Autodesk Inventor part; units mm, degrees
(part 3 of 6)
  line L1783 (-26.455, 14.4184) -> (-26.602, 14.5927)
  line L1784 (-26.602, 14.5927) -> (-26.7541, 14.7808)
  line L1785 (-26.7541, 14.7808) -> (-26.9091, 14.9811)
  line L1786 (-26.9091, 14.9811) -> (-27.041, 15.1586)
  arc A54 (-26.6482, 15.8389) -> (-27.041, 15.1586) centre (0, 0) ccw
  line L1787 (-26.6482, 15.8389) -> (-26.4285, 15.8134)
  line L1788 (-26.4285, 15.8134) -> (-26.1776, 15.7793)
  line L1789 (-26.1776, 15.7793) -> (-25.9387, 15.7417)
  line L1790 (-25.9387, 15.7417) -> (-25.7142, 15.7015)
  line L1791 (-25.7142, 15.7015) -> (-25.5018, 15.6589)
  line L1792 (-25.5018, 15.6589) -> (-25.3015, 15.6144)
  line L1793 (-25.3015, 15.6144) -> (-25.1161, 15.569)
  line L1794 (-25.1161, 15.569) -> (-24.9429, 15.5228)
  line L1795 (-24.9429, 15.5228) -> (-24.6058, 15.4237)
  line L1796 (-24.6058, 15.4237) -> (-24.5595, 15.4172)
  line L1797 (-24.5595, 15.4172) -> (-24.5238, 15.4191)
  line L1798 (-24.5238, 15.4191) -> (-24.4991, 15.4291)
  line L1799 (-24.4991, 15.4291) -> (-24.488, 15.4416)
  line L1800 (-24.488, 15.4416) -> (-24.2795, 15.7673)
  line L1801 (-24.2795, 15.7673) -> (-24.0668, 16.0903)
  line L1802 (-24.0668, 16.0903) -> (-24.0599, 16.1055)
  line L1803 (-24.0599, 16.1055) -> (-24.0608, 16.1321)
  line L1804 (-24.0608, 16.1321) -> (-24.0735, 16.1655)
  line L1805 (-24.0735, 16.1655) -> (-24.0984, 16.2052)
  line L1806 (-24.0984, 16.2052) -> (-24.326, 16.4728)
  line L1807 (-24.326, 16.4728) -> (-24.4386, 16.6122)
  line L1808 (-24.4386, 16.6122) -> (-24.5555, 16.7632)
  line L1809 (-24.5555, 16.7632) -> (-24.6777, 16.928)
  line L1810 (-24.6777, 16.928) -> (-24.8029, 17.1047)
  line L1811 (-24.8029, 17.1047) -> (-24.931, 17.2934)
  line L1812 (-24.931, 17.2934) -> (-25.0625, 17.4964)
  line L1813 (-25.0625, 17.4964) -> (-25.1957, 17.7118)
  line L1814 (-25.1957, 17.7118) -> (-25.3084, 17.9021)
  arc A55 (-24.8466, 18.5377) -> (-25.3084, 17.9021) centre (0, 0) ccw
  line L1815 (-24.8466, 18.5377) -> (-24.6308, 18.4893)
  line L1816 (-24.6308, 18.4893) -> (-24.3848, 18.4292)
  line L1817 (-24.3848, 18.4292) -> (-24.1511, 18.3668)
  line L1818 (-24.1511, 18.3668) -> (-23.932, 18.3034)
  line L1819 (-23.932, 18.3034) -> (-23.7253, 18.2388)
  line L1820 (-23.7253, 18.2388) -> (-23.5308, 18.1736)
  line L1821 (-23.5308, 18.1736) -> (-23.3511, 18.1091)
  line L1822 (-23.3511, 18.1091) -> (-23.1837, 18.045)
  line L1823 (-23.1837, 18.045) -> (-22.8588, 17.9112)
  line L1824 (-22.8588, 17.9112) -> (-22.8134, 17.8999)
  line L1825 (-22.8134, 17.8999) -> (-22.7777, 17.8981)
  line L1826 (-22.7777, 17.8981) -> (-22.7521, 17.9055)
  line L1827 (-22.7521, 17.9055) -> (-22.7398, 17.9167)
  line L1828 (-22.7398, 17.9167) -> (-22.4984, 18.2188)
  line L1829 (-22.4984, 18.2188) -> (-22.2531, 18.5178)
  line L1830 (-22.2531, 18.5178) -> (-22.2446, 18.5322)
  line L1831 (-22.2446, 18.5322) -> (-22.2427, 18.5587)
  line L1832 (-22.2427, 18.5587) -> (-22.2519, 18.5933)
  line L1833 (-22.2519, 18.5933) -> (-22.2724, 18.6353)
  line L1834 (-22.2724, 18.6353) -> (-22.4708, 18.9253)
  line L1835 (-22.4708, 18.9253) -> (-22.5683, 19.0757)
  line L1836 (-22.5683, 19.0757) -> (-22.6688, 19.2381)
  line L1837 (-22.6688, 19.2381) -> (-22.773, 19.4148)
  line L1838 (-22.773, 19.4148) -> (-22.8791, 19.6036)
  line L1839 (-22.8791, 19.6036) -> (-22.9867, 19.8047)
  line L1840 (-22.9867, 19.8047) -> (-23.0963, 20.0203)
  line L1841 (-23.0963, 20.0203) -> (-23.2063, 20.2484)
  line L1842 (-23.2063, 20.2484) -> (-23.2985, 20.4495)
  arc A56 (-22.7728, 21.0333) -> (-23.2985, 20.4495) centre (0, 0) ccw
  line L1843 (-22.7728, 21.0333) -> (-22.5632, 20.9626)
  line L1844 (-22.5632, 20.9626) -> (-22.3249, 20.8771)
  line L1845 (-22.3249, 20.8771) -> (-22.099, 20.7906)
  line L1846 (-22.099, 20.7906) -> (-21.8877, 20.7047)
  line L1847 (-21.8877, 20.7047) -> (-21.6889, 20.6189)
  line L1848 (-21.6889, 20.6189) -> (-21.5022, 20.5336)
  line L1849 (-21.5022, 20.5336) -> (-21.3302, 20.4507)
  line L1850 (-21.3302, 20.4507) -> (-21.1705, 20.3695)
  line L1851 (-21.1705, 20.3695) -> (-20.8614, 20.2025)
  line L1852 (-20.8614, 20.2025) -> (-20.8174, 20.1865)
  line L1853 (-20.8174, 20.1865) -> (-20.7821, 20.181)
  line L1854 (-20.7821, 20.181) -> (-20.7559, 20.1856)
  line L1855 (-20.7559, 20.1856) -> (-20.7424, 20.1955)
  line L1856 (-20.7424, 20.1955) -> (-20.4707, 20.4707)
  line L1857 (-20.4707, 20.4707) -> (-20.1955, 20.7424)
  line L1858 (-20.1955, 20.7424) -> (-20.1856, 20.7559)
  line L1859 (-20.1856, 20.7559) -> (-20.181, 20.7821)
  line L1860 (-20.181, 20.7821) -> (-20.1865, 20.8174)
  line L1861 (-20.1865, 20.8174) -> (-20.2025, 20.8614)
  line L1862 (-20.2025, 20.8614) -> (-20.3695, 21.1705)
  line L1863 (-20.3695, 21.1705) -> (-20.4507, 21.3302)
  line L1864 (-20.4507, 21.3302) -> (-20.5336, 21.5022)
  line L1865 (-20.5336, 21.5022) -> (-20.6189, 21.6889)
  line L1866 (-20.6189, 21.6889) -> (-20.7047, 21.8877)
  line L1867 (-20.7047, 21.8877) -> (-20.7906, 22.099)
  line L1868 (-20.7906, 22.099) -> (-20.8771, 22.3249)
  line L1869 (-20.8771, 22.3249) -> (-20.9626, 22.5632)
  line L1870 (-20.9626, 22.5632) -> (-21.0333, 22.7728)
  arc A57 (-20.4495, 23.2985) -> (-21.0333, 22.7728) centre (0, 0) ccw
  line L1871 (-20.4495, 23.2985) -> (-20.2484, 23.2063)
  line L1872 (-20.2484, 23.2063) -> (-20.0203, 23.0963)
  line L1873 (-20.0203, 23.0963) -> (-19.8047, 22.9867)
  line L1874 (-19.8047, 22.9867) -> (-19.6036, 22.8791)
  line L1875 (-19.6036, 22.8791) -> (-19.4148, 22.773)
  line L1876 (-19.4148, 22.773) -> (-19.2381, 22.6688)
  line L1877 (-19.2381, 22.6688) -> (-19.0757, 22.5683)
  line L1878 (-19.0757, 22.5683) -> (-18.9253, 22.4708)
  line L1879 (-18.9253, 22.4708) -> (-18.6353, 22.2724)
  line L1880 (-18.6353, 22.2724) -> (-18.5933, 22.2519)
  line L1881 (-18.5933, 22.2519) -> (-18.5587, 22.2427)
  line L1882 (-18.5587, 22.2427) -> (-18.5322, 22.2446)
  line L1883 (-18.5322, 22.2446) -> (-18.5178, 22.2531)
  line L1884 (-18.5178, 22.2531) -> (-18.2188, 22.4984)
  line L1885 (-18.2188, 22.4984) -> (-17.9167, 22.7398)
  line L1886 (-17.9167, 22.7398) -> (-17.9055, 22.7521)
  line L1887 (-17.9055, 22.7521) -> (-17.8981, 22.7777)
  line L1888 (-17.8981, 22.7777) -> (-17.8999, 22.8134)
  line L1889 (-17.8999, 22.8134) -> (-17.9112, 22.8588)
  line L1890 (-17.9112, 22.8588) -> (-18.045, 23.1837)
  line L1891 (-18.045, 23.1837) -> (-18.1091, 23.3511)
  line L1892 (-18.1091, 23.3511) -> (-18.1736, 23.5308)
  line L1893 (-18.1736, 23.5308) -> (-18.2388, 23.7253)
  line L1894 (-18.2388, 23.7253) -> (-18.3034, 23.932)
  line L1895 (-18.3034, 23.932) -> (-18.3668, 24.1511)
  line L1896 (-18.3668, 24.1511) -> (-18.4292, 24.3848)
  line L1897 (-18.4292, 24.3848) -> (-18.4893, 24.6308)
  line L1898 (-18.4893, 24.6308) -> (-18.5377, 24.8466)
  arc A58 (-17.9021, 25.3084) -> (-18.5377, 24.8466) centre (0, 0) ccw
  line L1899 (-17.9021, 25.3084) -> (-17.7118, 25.1957)
  line L1900 (-17.7118, 25.1957) -> (-17.4964, 25.0625)
  line L1901 (-17.4964, 25.0625) -> (-17.2934, 24.931)
  line L1902 (-17.2934, 24.931) -> (-17.1047, 24.8029)
  line L1903 (-17.1047, 24.8029) -> (-16.928, 24.6777)
  line L1904 (-16.928, 24.6777) -> (-16.7632, 24.5555)
  line L1905 (-16.7632, 24.5555) -> (-16.6122, 24.4386)
  line L1906 (-16.6122, 24.4386) -> (-16.4728, 24.326)
  line L1907 (-16.4728, 24.326) -> (-16.2052, 24.0984)
  line L1908 (-16.2052, 24.0984) -> (-16.1655, 24.0735)
  line L1909 (-16.1655, 24.0735) -> (-16.1321, 24.0608)
  line L1910 (-16.1321, 24.0608) -> (-16.1055, 24.0599)
  line L1911 (-16.1055, 24.0599) -> (-16.0903, 24.0668)
  line L1912 (-16.0903, 24.0668) -> (-15.7673, 24.2795)
  line L1913 (-15.7673, 24.2795) -> (-15.4416, 24.488)
  line L1914 (-15.4416, 24.488) -> (-15.4291, 24.4991)
  line L1915 (-15.4291, 24.4991) -> (-15.4191, 24.5238)
  line L1916 (-15.4191, 24.5238) -> (-15.4172, 24.5595)
  line L1917 (-15.4172, 24.5595) -> (-15.4237, 24.6058)
  line L1918 (-15.4237, 24.6058) -> (-15.5228, 24.9429)
  line L1919 (-15.5228, 24.9429) -> (-15.569, 25.1161)
  line L1920 (-15.569, 25.1161) -> (-15.6144, 25.3015)
  line L1921 (-15.6144, 25.3015) -> (-15.6589, 25.5018)
  line L1922 (-15.6589, 25.5018) -> (-15.7015, 25.7142)
  line L1923 (-15.7015, 25.7142) -> (-15.7417, 25.9387)
  line L1924 (-15.7417, 25.9387) -> (-15.7793, 26.1776)
  line L1925 (-15.7793, 26.1776) -> (-15.8134, 26.4285)
  line L1926 (-15.8134, 26.4285) -> (-15.8389, 26.6482)
  arc A59 (-15.1586, 27.041) -> (-15.8389, 26.6482) centre (0, 0) ccw
  line L1927 (-15.1586, 27.041) -> (-14.9811, 26.9091)
  line L1928 (-14.9811, 26.9091) -> (-14.7808, 26.7541)
  line L1929 (-14.7808, 26.7541) -> (-14.5927, 26.602)
  line L1930 (-14.5927, 26.602) -> (-14.4184, 26.455)
  line L1931 (-14.4184, 26.455) -> (-14.2558, 26.312)
  line L1932 (-14.2558, 26.312) -> (-14.1046, 26.1732)
  line L1933 (-14.1046, 26.1732) -> (-13.9666, 26.0412)
  line L1934 (-13.9666, 26.0412) -> (-13.8398, 25.9146)
  line L1935 (-13.8398, 25.9146) -> (-13.5974, 25.6603)
  line L1936 (-13.5974, 25.6603) -> (-13.5605, 25.6314)
  line L1937 (-13.5605, 25.6314) -> (-13.5287, 25.6153)
  line L1938 (-13.5287, 25.6153) -> (-13.5023, 25.6116)
  line L1939 (-13.5023, 25.6116) -> (-13.4865, 25.6168)
  line L1940 (-13.4865, 25.6168) -> (-13.143, 25.7946)
  line L1941 (-13.143, 25.7946) -> (-12.7973, 25.968)
  line L1942 (-12.7973, 25.968) -> (-12.7837, 25.9777)
  line L1943 (-12.7837, 25.9777) -> (-12.7712, 26.0012)
  line L1944 (-12.7712, 26.0012) -> (-12.7656, 26.0365)
  line L1945 (-12.7656, 26.0365) -> (-12.7672, 26.0833)
  line L1946 (-12.7672, 26.0833) -> (-12.8305, 26.4288)
  line L1947 (-12.8305, 26.4288) -> (-12.8584, 26.6059)
  line L1948 (-12.8584, 26.6059) -> (-12.8841, 26.7951)
  line L1949 (-12.8841, 26.7951) -> (-12.9075, 26.9989)
  line L1950 (-12.9075, 26.9989) -> (-12.9276, 27.2145)
  line L1951 (-12.9276, 27.2145) -> (-12.9441, 27.442)
  line L1952 (-12.9441, 27.442) -> (-12.9565, 27.6836)
  line L1953 (-12.9565, 27.6836) -> (-12.9642, 27.9367)
  line L1954 (-12.9642, 27.9367) -> (-12.9667, 28.1579)
  arc A60 (-12.249, 28.4774) -> (-12.9667, 28.1579) centre (0, 0) ccw
  line L1955 (-12.249, 28.4774) -> (-12.0862, 28.3276)
  line L1956 (-12.0862, 28.3276) -> (-11.9033, 28.1525)
  line L1957 (-11.9033, 28.1525) -> (-11.7321, 27.9817)
  line L1958 (-11.7321, 27.9817) -> (-11.5741, 27.8172)
  line L1959 (-11.5741, 27.8172) -> (-11.4273, 27.6579)
  line L1960 (-11.4273, 27.6579) -> (-11.2915, 27.5042)
  line L1961 (-11.2915, 27.5042) -> (-11.1681, 27.3584)
  line L1962 (-11.1681, 27.3584) -> (-11.0551, 27.2193)
  line L1963 (-11.0551, 27.2193) -> (-10.8407, 26.941)
  line L1964 (-10.8407, 26.941) -> (-10.807, 26.9085)
  line L1965 (-10.807, 26.9085) -> (-10.777, 26.8891)
  line L1966 (-10.777, 26.8891) -> (-10.7512, 26.8826)
  line L1967 (-10.7512, 26.8826) -> (-10.7349, 26.8862)
  line L1968 (-10.7349, 26.8862) -> (-10.3748, 27.0272)
  line L1969 (-10.3748, 27.0272) -> (-10.0128, 27.1634)
  line L1970 (-10.0128, 27.1634) -> (-9.9983, 27.1717)
  line L1971 (-9.9983, 27.1717) -> (-9.9834, 27.1937)
  line L1972 (-9.9834, 27.1937) -> (-9.9741, 27.2282)
  line L1973 (-9.9741, 27.2282) -> (-9.9708, 27.2749)
  line L1974 (-9.9708, 27.2749) -> (-9.9977, 27.6252)
  line L1975 (-9.9977, 27.6252) -> (-10.0069, 27.8042)
  line L1976 (-10.0069, 27.8042) -> (-10.0127, 27.995)
  line L1977 (-10.0127, 27.995) -> (-10.0146, 28.2002)
  line L1978 (-10.0146, 28.2002) -> (-10.0121, 28.4168)
  line L1979 (-10.0121, 28.4168) -> (-10.0047, 28.6447)
  line L1980 (-10.0047, 28.6447) -> (-9.9918, 28.8863)
  line L1981 (-9.9918, 28.8863) -> (-9.973, 29.1388)
  line L1982 (-9.973, 29.1388) -> (-9.9523, 29.359)
  arc A61 (-9.2052, 29.6018) -> (-9.9523, 29.359) centre (0, 0) ccw
  line L1983 (-9.2052, 29.6018) -> (-9.059, 29.4358)
  line L1984 (-9.059, 29.4358) -> (-8.8954, 29.2425)
  line L1985 (-8.8954, 29.2425) -> (-8.7429, 29.0547)
  line L1986 (-8.7429, 29.0547) -> (-8.603, 28.8746)
  line L1987 (-8.603, 28.8746) -> (-8.4737, 28.7009)
  line L1988 (-8.4737, 28.7009) -> (-8.3547, 28.5338)
  line L1989 (-8.3547, 28.5338) -> (-8.2472, 28.3759)
  line L1990 (-8.2472, 28.3759) -> (-8.1494, 28.2257)
  line L1991 (-8.1494, 28.2257) -> (-7.9652, 27.9266)
  line L1992 (-7.9652, 27.9266) -> (-7.9351, 27.8907)
  line L1993 (-7.9351, 27.8907) -> (-7.9073, 27.8683)
  line L1994 (-7.9073, 27.8683) -> (-7.8823, 27.8592)
  line L1995 (-7.8823, 27.8592) -> (-7.8657, 27.861)
  line L1996 (-7.8657, 27.861) -> (-7.4928, 27.9636)
  line L1997 (-7.4928, 27.9636) -> (-7.1186, 28.0612)
  line L1998 (-7.1186, 28.0612) -> (-7.1033, 28.0679)
  line L1999 (-7.1033, 28.0679) -> (-7.0862, 28.0883)
  line L2000 (-7.0862, 28.0883) -> (-7.0733, 28.1216)
  line L2001 (-7.0733, 28.1216) -> (-7.0652, 28.1677)
  line L2002 (-7.0652, 28.1677) -> (-7.0553, 28.5189)
  line L2003 (-7.0553, 28.5189) -> (-7.0457, 28.6979)
  line L2004 (-7.0457, 28.6979) -> (-7.0315, 28.8883)
  line L2005 (-7.0315, 28.8883) -> (-7.012, 29.0926)
  line L2006 (-7.012, 29.0926) -> (-6.9869, 29.3077)
  line L2007 (-6.9869, 29.3077) -> (-6.9557, 29.5336)
  line L2008 (-6.9557, 29.5336) -> (-6.9177, 29.7725)
  line L2009 (-6.9177, 29.7725) -> (-6.8726, 30.0216)
  line L2010 (-6.8726, 30.0216) -> (-6.829, 30.2385)
  arc A62 (-6.0605, 30.4018) -> (-6.829, 30.2385) centre (0, 0) ccw
  line L2011 (-6.0605, 30.4018) -> (-5.9325, 30.2214)
  line L2012 (-5.9325, 30.2214) -> (-5.79, 30.0122)
  line L2013 (-5.79, 30.0122) -> (-5.658, 29.8094)
  line L2014 (-5.658, 29.8094) -> (-5.5376, 29.6157)
  line L2015 (-5.5376, 29.6157) -> (-5.4272, 29.4294)
  line L2016 (-5.4272, 29.4294) -> (-5.3263, 29.2508)
  line L2017 (-5.3263, 29.2508) -> (-5.2359, 29.0826)
  line L2018 (-5.2359, 29.0826) -> (-5.1544, 28.9229)
  line L2019 (-5.1544, 28.9229) -> (-5.0025, 28.6062)
  line L2020 (-5.0025, 28.6062) -> (-4.9763, 28.5674)
  line L2021 (-4.9763, 28.5674) -> (-4.951, 28.5421)
  line L2022 (-4.951, 28.5421) -> (-4.927, 28.5305)
  line L2023 (-4.927, 28.5305) -> (-4.9104, 28.5306)
  line L2024 (-4.9104, 28.5306) -> (-4.5288, 28.5936)
  line L2025 (-4.5288, 28.5936) -> (-4.1464, 28.6516)
  line L2026 (-4.1464, 28.6516) -> (-4.1305, 28.6567)
  line L2027 (-4.1305, 28.6567) -> (-4.1114, 28.6751)
  line L2028 (-4.1114, 28.6751) -> (-4.0951, 28.7069)
  line L2029 (-4.0951, 28.7069) -> (-4.0822, 28.7519)
  line L2030 (-4.0822, 28.7519) -> (-4.0356, 29.1001)
  line L2031 (-4.0356, 29.1001) -> (-4.0074, 29.2771)
  line L2032 (-4.0074, 29.2771) -> (-3.9734, 29.465)
  line L2033 (-3.9734, 29.465) -> (-3.9326, 29.6661)
  line L2034 (-3.9326, 29.6661) -> (-3.8852, 29.8774)
  line L2035 (-3.8852, 29.8774) -> (-3.8305, 30.0989)
  line L2036 (-3.8305, 30.0989) -> (-3.7677, 30.3325)
  line L2037 (-3.7677, 30.3325) -> (-3.6968, 30.5755)
  line L2038 (-3.6968, 30.5755) -> (-3.6308, 30.7866)
  arc A63 (-2.8495, 30.8688) -> (-3.6308, 30.7866) centre (0, 0) ccw
  line L2039 (-2.8495, 30.8688) -> (-2.741, 30.676)
  line L2040 (-2.741, 30.676) -> (-2.6211, 30.453)
  line L2041 (-2.6211, 30.453) -> (-2.5111, 30.2376)
  line L2042 (-2.5111, 30.2376) -> (-2.4116, 30.0323)
  line L2043 (-2.4116, 30.0323) -> (-2.3213, 29.8355)
  line L2044 (-2.3213, 29.8355) -> (-2.2396, 29.6473)
  line L2045 (-2.2396, 29.6473) -> (-2.1673, 29.4705)
  line L2046 (-2.1673, 29.4705) -> (-2.1029, 29.3033)
  line L2047 (-2.1029, 29.3033) -> (-1.9849, 28.9724)
  line L2048 (-1.9849, 28.9724) -> (-1.9629, 28.931)
  line L2049 (-1.9629, 28.931) -> (-1.9404, 28.9033)
  line L2050 (-1.9404, 28.9033) -> (-1.9178, 28.8892)
  line L2051 (-1.9178, 28.8892) -> (-1.9012, 28.8876)
  line L2052 (-1.9012, 28.8876) -> (-1.5151, 28.9103)
  line L2053 (-1.5151, 28.9103) -> (-1.1288, 28.9281)
  line L2054 (-1.1288, 28.9281) -> (-1.1124, 28.9314)
  line L2055 (-1.1124, 28.9314) -> (-1.0915, 28.9478)
  line L2056 (-1.0915, 28.9478) -> (-1.0719, 28.9777)
  line L2057 (-1.0719, 28.9777) -> (-1.0544, 29.0211)
  line L2058 (-1.0544, 29.0211) -> (-0.9717, 29.3626)
  line L2059 (-0.9717, 29.3626) -> (-0.9251, 29.5356)
  line L2060 (-0.9251, 29.5356) -> (-0.8717, 29.719)
  line L2061 (-0.8717, 29.719) -> (-0.8101, 29.9147)
  line L2062 (-0.8101, 29.9147) -> (-0.7408, 30.1199)
  line L2063 (-0.7408, 30.1199) -> (-0.6634, 30.3344)
  line L2064 (-0.6634, 30.3344) -> (-0.5765, 30.5601)
  line L2065 (-0.5765, 30.5601) -> (-0.4805, 30.7945)
  line L2066 (-0.4805, 30.7945) -> (-0.3928, 30.9975)
  arc A64 (0.3928, 30.9975) -> (-0.3928, 30.9975) centre (0, 0) ccw
  line L2067 (0.3928, 30.9975) -> (0.4805, 30.7945)
  line L2068 (0.4805, 30.7945) -> (0.5765, 30.5601)
  line L2069 (0.5765, 30.5601) -> (0.6634, 30.3344)
  line L2070 (0.6634, 30.3344) -> (0.7408, 30.1199)
  line L2071 (0.7408, 30.1199) -> (0.8101, 29.9147)
  line L2072 (0.8101, 29.9147) -> (0.8717, 29.719)
  line L2073 (0.8717, 29.719) -> (0.9251, 29.5356)
  line L2074 (0.9251, 29.5356) -> (0.9717, 29.3626)
  line L2075 (0.9717, 29.3626) -> (1.0544, 29.0211)
  line L2076 (1.0544, 29.0211) -> (1.0719, 28.9777)
  line L2077 (1.0719, 28.9777) -> (1.0915, 28.9478)
  line L2078 (1.0915, 28.9478) -> (1.1124, 28.9314)
  line L2079 (1.1124, 28.9314) -> (1.1288, 28.9281)
  line L2080 (1.1288, 28.9281) -> (1.5151, 28.9103)
  line L2081 (1.5151, 28.9103) -> (1.9012, 28.8876)
  line L2082 (1.9012, 28.8876) -> (1.9178, 28.8892)
  line L2083 (1.9178, 28.8892) -> (1.9404, 28.9033)
  line L2084 (1.9404, 28.9033) -> (1.9629, 28.931)
  line L2085 (1.9629, 28.931) -> (1.9849, 28.9724)
  line L2086 (1.9849, 28.9724) -> (2.1029, 29.3033)
  line L2087 (2.1029, 29.3033) -> (2.1673, 29.4705)
  line L2088 (2.1673, 29.4705) -> (2.2396, 29.6473)
  line L2089 (2.2396, 29.6473) -> (2.3213, 29.8355)
  line L2090 (2.3213, 29.8355) -> (2.4116, 30.0323)
  line L2091 (2.4116, 30.0323) -> (2.5111, 30.2376)
  line L2092 (2.5111, 30.2376) -> (2.6211, 30.453)
  line L2093 (2.6211, 30.453) -> (2.741, 30.676)
  line L2094 (2.741, 30.676) -> (2.8495, 30.8688)
  arc A65 (3.6308, 30.7866) -> (2.8495, 30.8688) centre (0, 0) ccw
  line L2095 (3.6308, 30.7866) -> (3.6968, 30.5755)
  line L2096 (3.6968, 30.5755) -> (3.7677, 30.3325)
  line L2097 (3.7677, 30.3325) -> (3.8305, 30.0989)
  line L2098 (3.8305, 30.0989) -> (3.8852, 29.8774)
  line L2099 (3.8852, 29.8774) -> (3.9326, 29.6661)
  line L2100 (3.9326, 29.6661) -> (3.9734, 29.465)
  line L2101 (3.9734, 29.465) -> (4.0074, 29.2771)
  line L2102 (4.0074, 29.2771) -> (4.0356, 29.1001)
  line L2103 (4.0356, 29.1001) -> (4.0822, 28.7519)
  line L2104 (4.0822, 28.7519) -> (4.0951, 28.7069)
  line L2105 (4.0951, 28.7069) -> (4.1114, 28.6751)
  line L2106 (4.1114, 28.6751) -> (4.1305, 28.6567)
  line L2107 (4.1305, 28.6567) -> (4.1464, 28.6516)
  line L2108 (4.1464, 28.6516) -> (4.5288, 28.5936)
  line L2109 (4.5288, 28.5936) -> (4.9104, 28.5306)
  line L2110 (4.9104, 28.5306) -> (4.927, 28.5305)
  line L2111 (4.927, 28.5305) -> (4.951, 28.5421)
  line L2112 (4.951, 28.5421) -> (4.9763, 28.5674)
  line L2113 (4.9763, 28.5674) -> (5.0025, 28.6062)
  line L2114 (5.0025, 28.6062) -> (5.1544, 28.9229)
  line L2115 (5.1544, 28.9229) -> (5.2359, 29.0826)
  line L2116 (5.2359, 29.0826) -> (5.3263, 29.2508)
  line L2117 (5.3263, 29.2508) -> (5.4272, 29.4294)
  line L2118 (5.4272, 29.4294) -> (5.5376, 29.6157)
  line L2119 (5.5376, 29.6157) -> (5.658, 29.8094)
  line L2120 (5.658, 29.8094) -> (5.79, 30.0122)
  line L2121 (5.79, 30.0122) -> (5.9325, 30.2214)
  line L2122 (5.9325, 30.2214) -> (6.0605, 30.4018)
  arc A66 (6.829, 30.2385) -> (6.0605, 30.4018) centre (0, 0) ccw
  line L2123 (6.829, 30.2385) -> (6.8726, 30.0216)
  line L2124 (6.8726, 30.0216) -> (6.9177, 29.7725)
  line L2125 (6.9177, 29.7725) -> (6.9557, 29.5336)
  line L2126 (6.9557, 29.5336) -> (6.9869, 29.3077)
  line L2127 (6.9869, 29.3077) -> (7.012, 29.0926)
  line L2128 (7.012, 29.0926) -> (7.0315, 28.8883)
  line L2129 (7.0315, 28.8883) -> (7.0457, 28.6979)
  line L2130 (7.0457, 28.6979) -> (7.0553, 28.5189)
  line L2131 (7.0553, 28.5189) -> (7.0652, 28.1677)
  line L2132 (7.0652, 28.1677) -> (7.0733, 28.1216)
  line L2133 (7.0733, 28.1216) -> (7.0862, 28.0883)
  line L2134 (7.0862, 28.0883) -> (7.1033, 28.0679)
  line L2135 (7.1033, 28.0679) -> (7.1186, 28.0612)
  line L2136 (7.1186, 28.0612) -> (7.4928, 27.9636)
  line L2137 (7.4928, 27.9636) -> (7.8657, 27.861)
  line L2138 (7.8657, 27.861) -> (7.8823, 27.8592)
  line L2139 (7.8823, 27.8592) -> (7.9073, 27.8683)
  line L2140 (7.9073, 27.8683) -> (7.9351, 27.8907)
  line L2141 (7.9351, 27.8907) -> (7.9652, 27.9266)
  line L2142 (7.9652, 27.9266) -> (8.1494, 28.2257)
  line L2143 (8.1494, 28.2257) -> (8.2472, 28.3759)
  line L2144 (8.2472, 28.3759) -> (8.3547, 28.5338)
  line L2145 (8.3547, 28.5338) -> (8.4737, 28.7009)
  line L2146 (8.4737, 28.7009) -> (8.603, 28.8746)
  line L2147 (8.603, 28.8746) -> (8.7429, 29.0547)
  line L2148 (8.7429, 29.0547) -> (8.8954, 29.2425)
  line L2149 (8.8954, 29.2425) -> (9.059, 29.4358)
  line L2150 (9.059, 29.4358) -> (9.2052, 29.6018)
  arc A67 (9.9523, 29.359) -> (9.2052, 29.6018) centre (0, 0) ccw
  line L2151 (9.9523, 29.359) -> (9.973, 29.1388)
  line L2152 (9.973, 29.1388) -> (9.9918, 28.8863)
  line L2153 (9.9918, 28.8863) -> (10.0047, 28.6447)
  line L2154 (10.0047, 28.6447) -> (10.0121, 28.4168)
  line L2155 (10.0121, 28.4168) -> (10.0146, 28.2002)
  line L2156 (10.0146, 28.2002) -> (10.0127, 27.995)
  line L2157 (10.0127, 27.995) -> (10.0069, 27.8042)
  line L2158 (10.0069, 27.8042) -> (9.9977, 27.6252)
  line L2159 (9.9977, 27.6252) -> (9.9708, 27.2749)
  line L2160 (9.9708, 27.2749) -> (9.9741, 27.2282)
  line L2161 (9.9741, 27.2282) -> (9.9834, 27.1937)
  line L2162 (9.9834, 27.1937) -> (9.9983, 27.1717)
  line L2163 (9.9983, 27.1717) -> (10.0128, 27.1634)
  line L2164 (10.0128, 27.1634) -> (10.3748, 27.0272)
  line L2165 (10.3748, 27.0272) -> (10.7349, 26.8862)
  line L2166 (10.7349, 26.8862) -> (10.7512, 26.8826)
  line L2167 (10.7512, 26.8826) -> (10.777, 26.8891)
  line L2168 (10.777, 26.8891) -> (10.807, 26.9085)
  line L2169 (10.807, 26.9085) -> (10.8407, 26.941)
  line L2170 (10.8407, 26.941) -> (11.0551, 27.2193)
  line L2171 (11.0551, 27.2193) -> (11.1681, 27.3584)
  line L2172 (11.1681, 27.3584) -> (11.2915, 27.5042)
  line L2173 (11.2915, 27.5042) -> (11.4273, 27.6579)
  line L2174 (11.4273, 27.6579) -> (11.5741, 27.8172)
  line L2175 (11.5741, 27.8172) -> (11.7321, 27.9817)
  line L2176 (11.7321, 27.9817) -> (11.9033, 28.1525)
  line L2177 (11.9033, 28.1525) -> (12.0862, 28.3276)
  line L2178 (12.0862, 28.3276) -> (12.249, 28.4774)
  arc A68 (12.9667, 28.1579) -> (12.249, 28.4774) centre (0, 0) ccw
  line L2179 (12.9667, 28.1579) -> (12.9642, 27.9367)
  line L2180 (12.9642, 27.9367) -> (12.9565, 27.6836)
  line L2181 (12.9565, 27.6836) -> (12.9441, 27.442)
  line L2182 (12.9441, 27.442) -> (12.9276, 27.2145)
  line L2183 (12.9276, 27.2145) -> (12.9075, 26.9989)
  line L2184 (12.9075, 26.9989) -> (12.8841, 26.7951)
  line L2185 (12.8841, 26.7951) -> (12.8584, 26.6059)
  line L2186 (12.8584, 26.6059) -> (12.8305, 26.4288)
  line L2187 (12.8305, 26.4288) -> (12.7672, 26.0833)
  line L2188 (12.7672, 26.0833) -> (12.7656, 26.0365)
  line L2189 (12.7656, 26.0365) -> (12.7712, 26.0012)
  line L2190 (12.7712, 26.0012) -> (12.7837, 25.9777)
  line L2191 (12.7837, 25.9777) -> (12.7973, 25.968)
  line L2192 (12.7973, 25.968) -> (13.143, 25.7946)
  line L2193 (13.143, 25.7946) -> (13.4865, 25.6168)
  line L2194 (13.4865, 25.6168) -> (13.5023, 25.6116)
  line L2195 (13.5023, 25.6116) -> (13.5287, 25.6153)
  line L2196 (13.5287, 25.6153) -> (13.5605, 25.6314)
  line L2197 (13.5605, 25.6314) -> (13.5974, 25.6603)
  line L2198 (13.5974, 25.6603) -> (13.8398, 25.9146)
  line L2199 (13.8398, 25.9146) -> (13.9666, 26.0412)
  line L2200 (13.9666, 26.0412) -> (14.1046, 26.1732)
  line L2201 (14.1046, 26.1732) -> (14.2558, 26.312)
  line L2202 (14.2558, 26.312) -> (14.4184, 26.455)
  line L2203 (14.4184, 26.455) -> (14.5927, 26.602)
  line L2204 (14.5927, 26.602) -> (14.7808, 26.7541)
  line L2205 (14.7808, 26.7541) -> (14.9811, 26.9091)
  line L2206 (14.9811, 26.9091) -> (15.1586, 27.041)
  arc A69 (15.8389, 26.6482) -> (15.1586, 27.041) centre (0, 0) ccw
  line L2207 (15.8389, 26.6482) -> (15.8134, 26.4285)
  line L2208 (15.8134, 26.4285) -> (15.7793, 26.1776)
  line L2209 (15.7793, 26.1776) -> (15.7417, 25.9387)
  line L2210 (15.7417, 25.9387) -> (15.7015, 25.7142)
  line L2211 (15.7015, 25.7142) -> (15.6589, 25.5018)
  line L2212 (15.6589, 25.5018) -> (15.6144, 25.3015)
  line L2213 (15.6144, 25.3015) -> (15.569, 25.1161)
  line L2214 (15.569, 25.1161) -> (15.5228, 24.9429)
  line L2215 (15.5228, 24.9429) -> (15.4237, 24.6058)
  line L2216 (15.4237, 24.6058) -> (15.4172, 24.5595)
  line L2217 (15.4172, 24.5595) -> (15.4191, 24.5238)
  line L2218 (15.4191, 24.5238) -> (15.4291, 24.4991)
  line L2219 (15.4291, 24.4991) -> (15.4416, 24.488)
  line L2220 (15.4416, 24.488) -> (15.7673, 24.2795)
  line L2221 (15.7673, 24.2795) -> (16.0903, 24.0668)
  line L2222 (16.0903, 24.0668) -> (16.1055, 24.0599)
  line L2223 (16.1055, 24.0599) -> (16.1321, 24.0608)
  line L2224 (16.1321, 24.0608) -> (16.1655, 24.0735)
  line L2225 (16.1655, 24.0735) -> (16.2052, 24.0984)
  line L2226 (16.2052, 24.0984) -> (16.4728, 24.326)
  line L2227 (16.4728, 24.326) -> (16.6122, 24.4386)
  line L2228 (16.6122, 24.4386) -> (16.7632, 24.5555)
  line L2229 (16.7632, 24.5555) -> (16.928, 24.6777)
  line L2230 (16.928, 24.6777) -> (17.1047, 24.8029)
  line L2231 (17.1047, 24.8029) -> (17.2934, 24.931)
  line L2232 (17.2934, 24.931) -> (17.4964, 25.0625)
  line L2233 (17.4964, 25.0625) -> (17.7118, 25.1957)
  line L2234 (17.7118, 25.1957) -> (17.9021, 25.3084)
  arc A70 (18.5377, 24.8466) -> (17.9021, 25.3084) centre (0, 0) ccw
  line L2235 (18.5377, 24.8466) -> (18.4893, 24.6308)
  line L2236 (18.4893, 24.6308) -> (18.4292, 24.3848)
  line L2237 (18.4292, 24.3848) -> (18.3668, 24.1511)
  line L2238 (18.3668, 24.1511) -> (18.3034, 23.932)
  line L2239 (18.3034, 23.932) -> (18.2388, 23.7253)
  line L2240 (18.2388, 23.7253) -> (18.1736, 23.5308)
  line L2241 (18.1736, 23.5308) -> (18.1091, 23.3511)
  line L2242 (18.1091, 23.3511) -> (18.045, 23.1837)
  line L2243 (18.045, 23.1837) -> (17.9112, 22.8588)
  line L2244 (17.9112, 22.8588) -> (17.8999, 22.8134)
  line L2245 (17.8999, 22.8134) -> (17.8981, 22.7777)
  line L2246 (17.8981, 22.7777) -> (17.9055, 22.7521)
  line L2247 (17.9055, 22.7521) -> (17.9167, 22.7398)
  line L2248 (17.9167, 22.7398) -> (18.2188, 22.4984)
  line L2249 (18.2188, 22.4984) -> (18.5178, 22.2531)
  line L2250 (18.5178, 22.2531) -> (18.5322, 22.2446)
  line L2251 (18.5322, 22.2446) -> (18.5587, 22.2427)
  line L2252 (18.5587, 22.2427) -> (18.5933, 22.2519)
  line L2253 (18.5933, 22.2519) -> (18.6353, 22.2724)
  line L2254 (18.6353, 22.2724) -> (18.9253, 22.4708)
  line L2255 (18.9253, 22.4708) -> (19.0757, 22.5683)
  line L2256 (19.0757, 22.5683) -> (19.2381, 22.6688)
  line L2257 (19.2381, 22.6688) -> (19.4148, 22.773)
  line L2258 (19.4148, 22.773) -> (19.6036, 22.8791)
  line L2259 (19.6036, 22.8791) -> (19.8047, 22.9867)
  line L2260 (19.8047, 22.9867) -> (20.0203, 23.0963)
  line L2261 (20.0203, 23.0963) -> (20.2484, 23.2063)
  line L2262 (20.2484, 23.2063) -> (20.4495, 23.2985)
  arc A71 (21.0333, 22.7728) -> (20.4495, 23.2985) centre (0, 0) ccw
  line L2263 (21.0333, 22.7728) -> (20.9626, 22.5632)
  line L2264 (20.9626, 22.5632) -> (20.8771, 22.3249)
  line L2265 (20.8771, 22.3249) -> (20.7906, 22.099)
  line L2266 (20.7906, 22.099) -> (20.7047, 21.8877)
  line L2267 (20.7047, 21.8877) -> (20.6189, 21.6889)
  line L2268 (20.6189, 21.6889) -> (20.5336, 21.5022)
  line L2269 (20.5336, 21.5022) -> (20.4507, 21.3302)
  line L2270 (20.4507, 21.3302) -> (20.3695, 21.1705)
  line L2271 (20.3695, 21.1705) -> (20.2025, 20.8614)
  line L2272 (20.2025, 20.8614) -> (20.1865, 20.8174)
  line L2273 (20.1865, 20.8174) -> (20.181, 20.7821)
  line L2274 (20.181, 20.7821) -> (20.1856, 20.7559)
  line L2275 (20.1856, 20.7559) -> (20.1955, 20.7424)
  line L2276 (20.1955, 20.7424) -> (20.4707, 20.4707)
  line L2277 (20.4707, 20.4707) -> (20.7424, 20.1955)
  line L2278 (20.7424, 20.1955) -> (20.7559, 20.1856)
  line L2279 (20.7559, 20.1856) -> (20.7821, 20.181)
  line L2280 (20.7821, 20.181) -> (20.8174, 20.1865)
  line L2281 (20.8174, 20.1865) -> (20.8614, 20.2025)
  line L2282 (20.8614, 20.2025) -> (21.1705, 20.3695)
  line L2283 (21.1705, 20.3695) -> (21.3302, 20.4507)
  line L2284 (21.3302, 20.4507) -> (21.5022, 20.5336)
  line L2285 (21.5022, 20.5336) -> (21.6889, 20.6189)
  line L2286 (21.6889, 20.6189) -> (21.8877, 20.7047)
  line L2287 (21.8877, 20.7047) -> (22.099, 20.7906)
  line L2288 (22.099, 20.7906) -> (22.3249, 20.8771)
  line L2289 (22.3249, 20.8771) -> (22.5632, 20.9626)
  line L2290 (22.5632, 20.9626) -> (22.7728, 21.0333)
  arc A72 (23.2985, 20.4495) -> (22.7728, 21.0333) centre (0, 0) ccw
  line L2291 (23.2985, 20.4495) -> (23.2063, 20.2484)
  line L2292 (23.2063, 20.2484) -> (23.0963, 20.0203)
  line L2293 (23.0963, 20.0203) -> (22.9867, 19.8047)
  line L2294 (22.9867, 19.8047) -> (22.8791, 19.6036)
  line L2295 (22.8791, 19.6036) -> (22.773, 19.4148)
  line L2296 (22.773, 19.4148) -> (22.6688, 19.2381)
  line L2297 (22.6688, 19.2381) -> (22.5683, 19.0757)
  line L2298 (22.5683, 19.0757) -> (22.4708, 18.9253)
  line L2299 (22.4708, 18.9253) -> (22.2724, 18.6353)
  line L2300 (22.2724, 18.6353) -> (22.2519, 18.5933)
  line L2301 (22.2519, 18.5933) -> (22.2427, 18.5587)
  line L2302 (22.2427, 18.5587) -> (22.2446, 18.5322)
  line L2303 (22.2446, 18.5322) -> (22.2531, 18.5178)
  line L2304 (22.2531, 18.5178) -> (22.4984, 18.2188)
  line L2305 (22.4984, 18.2188) -> (22.7398, 17.9167)
  line L2306 (22.7398, 17.9167) -> (22.7521, 17.9055)
  line L2307 (22.7521, 17.9055) -> (22.7777, 17.8981)
  line L2308 (22.7777, 17.8981) -> (22.8134, 17.8999)
  line L2309 (22.8134, 17.8999) -> (22.8588, 17.9112)
  line L2310 (22.8588, 17.9112) -> (23.1837, 18.045)
  line L2311 (23.1837, 18.045) -> (23.3511, 18.1091)
  line L2312 (23.3511, 18.1091) -> (23.5308, 18.1736)
  line L2313 (23.5308, 18.1736) -> (23.7253, 18.2388)
  line L2314 (23.7253, 18.2388) -> (23.932, 18.3034)
  line L2315 (23.932, 18.3034) -> (24.1511, 18.3668)
  line L2316 (24.1511, 18.3668) -> (24.3848, 18.4292)
  line L2317 (24.3848, 18.4292) -> (24.6308, 18.4893)
  line L2318 (24.6308, 18.4893) -> (24.8466, 18.5377)
  arc A73 (25.3084, 17.9021) -> (24.8466, 18.5377) centre (0, 0) ccw
  line L2319 (25.3084, 17.9021) -> (25.1957, 17.7118)
  line L2320 (25.1957, 17.7118) -> (25.0625, 17.4964)
  line L2321 (25.0625, 17.4964) -> (24.931, 17.2934)
  line L2322 (24.931, 17.2934) -> (24.8029, 17.1047)
  line L2323 (24.8029, 17.1047) -> (24.6777, 16.928)
  line L2324 (24.6777, 16.928) -> (24.5555, 16.7632)
  line L2325 (24.5555, 16.7632) -> (24.4386, 16.6122)
  line L2326 (24.4386, 16.6122) -> (24.326, 16.4728)
  line L2327 (24.326, 16.4728) -> (24.0984, 16.2052)
  line L2328 (24.0984, 16.2052) -> (24.0735, 16.1655)
  line L2329 (24.0735, 16.1655) -> (24.0608, 16.1321)
  line L2330 (24.0608, 16.1321) -> (24.0599, 16.1055)
  line L2331 (24.0599, 16.1055) -> (24.0668, 16.0903)
  line L2332 (24.0668, 16.0903) -> (24.2795, 15.7673)
  line L2333 (24.2795, 15.7673) -> (24.488, 15.4416)
  line L2334 (24.488, 15.4416) -> (24.4991, 15.4291)
  line L2335 (24.4991, 15.4291) -> (24.5238, 15.4191)
  line L2336 (24.5238, 15.4191) -> (24.5595, 15.4172)
  line L2337 (24.5595, 15.4172) -> (24.6058, 15.4237)
  line L2338 (24.6058, 15.4237) -> (24.9429, 15.5228)
  line L2339 (24.9429, 15.5228) -> (25.1161, 15.569)
  line L2340 (25.1161, 15.569) -> (25.3015, 15.6144)
  line L2341 (25.3015, 15.6144) -> (25.5018, 15.6589)
  line L2342 (25.5018, 15.6589) -> (25.7142, 15.7015)
  line L2343 (25.7142, 15.7015) -> (25.9387, 15.7417)
  line L2344 (25.9387, 15.7417) -> (26.1776, 15.7793)
  line L2345 (26.1776, 15.7793) -> (26.4285, 15.8134)
  line L2346 (26.4285, 15.8134) -> (26.6482, 15.8389)
  arc A74 (27.041, 15.1586) -> (26.6482, 15.8389) centre (0, 0) ccw
  line L2347 (27.041, 15.1586) -> (26.9091, 14.9811)
  line L2348 (26.9091, 14.9811) -> (26.7541, 14.7808)
  line L2349 (26.7541, 14.7808) -> (26.602, 14.5927)
  line L2350 (26.602, 14.5927) -> (26.455, 14.4184)
  line L2351 (26.455, 14.4184) -> (26.312, 14.2558)
  line L2352 (26.312, 14.2558) -> (26.1732, 14.1046)
  line L2353 (26.1732, 14.1046) -> (26.0412, 13.9666)
  line L2354 (26.0412, 13.9666) -> (25.9146, 13.8398)
  line L2355 (25.9146, 13.8398) -> (25.6603, 13.5974)
  line L2356 (25.6603, 13.5974) -> (25.6314, 13.5605)
  line L2357 (25.6314, 13.5605) -> (25.6153, 13.5287)
  line L2358 (25.6153, 13.5287) -> (25.6116, 13.5023)
  line L2359 (25.6116, 13.5023) -> (25.6168, 13.4865)
  line L2360 (25.6168, 13.4865) -> (25.7946, 13.143)
  line L2361 (25.7946, 13.143) -> (25.968, 12.7973)
  line L2362 (25.968, 12.7973) -> (25.9777, 12.7837)
  line L2363 (25.9777, 12.7837) -> (26.0012, 12.7712)
  line L2364 (26.0012, 12.7712) -> (26.0365, 12.7656)
  line L2365 (26.0365, 12.7656) -> (26.0833, 12.7672)
  line L2366 (26.0833, 12.7672) -> (26.4288, 12.8305)
  line L2367 (26.4288, 12.8305) -> (26.6059, 12.8584)
  line L2368 (26.6059, 12.8584) -> (26.7951, 12.8841)
  line L2369 (26.7951, 12.8841) -> (26.9989, 12.9075)
  line L2370 (26.9989, 12.9075) -> (27.2145, 12.9276)
  line L2371 (27.2145, 12.9276) -> (27.442, 12.9441)
  line L2372 (27.442, 12.9441) -> (27.6836, 12.9565)
  line L2373 (27.6836, 12.9565) -> (27.9367, 12.9642)
  line L2374 (27.9367, 12.9642) -> (28.1579, 12.9667)
  arc A75 (28.4774, 12.249) -> (28.1579, 12.9667) centre (0, 0) ccw
  line L2375 (28.4774, 12.249) -> (28.3276, 12.0862)
  line L2376 (28.3276, 12.0862) -> (28.1525, 11.9033)
  line L2377 (28.1525, 11.9033) -> (27.9817, 11.7321)
  line L2378 (27.9817, 11.7321) -> (27.8172, 11.5741)
  line L2379 (27.8172, 11.5741) -> (27.6579, 11.4273)
  line L2380 (27.6579, 11.4273) -> (27.5042, 11.2915)
  line L2381 (27.5042, 11.2915) -> (27.3584, 11.1681)
  line L2382 (27.3584, 11.1681) -> (27.2193, 11.0551)
  line L2383 (27.2193, 11.0551) -> (26.941, 10.8407)
  line L2384 (26.941, 10.8407) -> (26.9085, 10.807)
  line L2385 (26.9085, 10.807) -> (26.8891, 10.777)
  line L2386 (26.8891, 10.777) -> (26.8826, 10.7512)
  line L2387 (26.8826, 10.7512) -> (26.8862, 10.7349)
  line L2388 (26.8862, 10.7349) -> (27.0272, 10.3748)
  line L2389 (27.0272, 10.3748) -> (27.1634, 10.0128)
  line L2390 (27.1634, 10.0128) -> (27.1717, 9.9983)
  line L2391 (27.1717, 9.9983) -> (27.1937, 9.9834)
  line L2392 (27.1937, 9.9834) -> (27.2282, 9.9741)
  line L2393 (27.2282, 9.9741) -> (27.2749, 9.9708)
  line L2394 (27.2749, 9.9708) -> (27.6252, 9.9977)
  line L2395 (27.6252, 9.9977) -> (27.8042, 10.0069)
  line L2396 (27.8042, 10.0069) -> (27.995, 10.0127)
  line L2397 (27.995, 10.0127) -> (28.2002, 10.0146)
  line L2398 (28.2002, 10.0146) -> (28.4168, 10.0121)
  line L2399 (28.4168, 10.0121) -> (28.6447, 10.0047)
  line L2400 (28.6447, 10.0047) -> (28.8863, 9.9918)
  line L2401 (28.8863, 9.9918) -> (29.1388, 9.973)
  line L2402 (29.1388, 9.973) -> (29.359, 9.9523)
  arc A76 (29.6018, 9.2052) -> (29.359, 9.9523) centre (0, 0) ccw
  line L2403 (29.6018, 9.2052) -> (29.4358, 9.059)
  line L2404 (29.4358, 9.059) -> (29.2425, 8.8954)
  line L2405 (29.2425, 8.8954) -> (29.0547, 8.7429)
  line L2406 (29.0547, 8.7429) -> (28.8746, 8.603)
  line L2407 (28.8746, 8.603) -> (28.7009, 8.4737)
  line L2408 (28.7009, 8.4737) -> (28.5338, 8.3547)
  line L2409 (28.5338, 8.3547) -> (28.3759, 8.2472)
  line L2410 (28.3759, 8.2472) -> (28.2257, 8.1494)
  line L2411 (28.2257, 8.1494) -> (27.9266, 7.9652)
  line L2412 (27.9266, 7.9652) -> (27.8907, 7.9351)
  line L2413 (27.8907, 7.9351) -> (27.8683, 7.9073)
  line L2414 (27.8683, 7.9073) -> (27.8592, 7.8823)
  line L2415 (27.8592, 7.8823) -> (27.861, 7.8657)
  line L2416 (27.861, 7.8657) -> (27.9636, 7.4928)
  line L2417 (27.9636, 7.4928) -> (28.0612, 7.1186)
  line L2418 (28.0612, 7.1186) -> (28.0679, 7.1033)
  line L2419 (28.0679, 7.1033) -> (28.0883, 7.0862)
  line L2420 (28.0883, 7.0862) -> (28.1216, 7.0733)
  line L2421 (28.1216, 7.0733) -> (28.1677, 7.0652)
  line L2422 (28.1677, 7.0652) -> (28.5189, 7.0553)
  line L2423 (28.5189, 7.0553) -> (28.6979, 7.0457)
  line L2424 (28.6979, 7.0457) -> (28.8883, 7.0315)
  line L2425 (28.8883, 7.0315) -> (29.0926, 7.012)
  line L2426 (29.0926, 7.012) -> (29.3077, 6.9869)
  line L2427 (29.3077, 6.9869) -> (29.5336, 6.9557)
  line L2428 (29.5336, 6.9557) -> (29.7725, 6.9177)
  line L2429 (29.7725, 6.9177) -> (30.0216, 6.8726)
  line L2430 (30.0216, 6.8726) -> (30.2385, 6.829)
  arc A77 (30.4018, 6.0605) -> (30.2385, 6.829) centre (0, 0) ccw
  line L2431 (30.4018, 6.0605) -> (30.2214, 5.9325)
  line L2432 (30.2214, 5.9325) -> (30.0122, 5.79)
  line L2433 (30.0122, 5.79) -> (29.8094, 5.658)
  line L2434 (29.8094, 5.658) -> (29.6157, 5.5376)
  line L2435 (29.6157, 5.5376) -> (29.4294, 5.4272)
  line L2436 (29.4294, 5.4272) -> (29.2508, 5.3263)
  line L2437 (29.2508, 5.3263) -> (29.0826, 5.2359)
  line L2438 (29.0826, 5.2359) -> (28.9229, 5.1544)
  line L2439 (28.9229, 5.1544) -> (28.6062, 5.0025)
  line L2440 (28.6062, 5.0025) -> (28.5674, 4.9763)
  line L2441 (28.5674, 4.9763) -> (28.5421, 4.951)
  line L2442 (28.5421, 4.951) -> (28.5305, 4.927)
  line L2443 (28.5305, 4.927) -> (28.5306, 4.9104)
  line L2444 (28.5306, 4.9104) -> (28.5936, 4.5288)
  line L2445 (28.5936, 4.5288) -> (28.6516, 4.1464)
  line L2446 (28.6516, 4.1464) -> (28.6567, 4.1305)
  line L2447 (28.6567, 4.1305) -> (28.6751, 4.1114)
  line L2448 (28.6751, 4.1114) -> (28.7069, 4.0951)
  line L2449 (28.7069, 4.0951) -> (28.7519, 4.0822)
  line L2450 (28.7519, 4.0822) -> (29.1001, 4.0356)
  line L2451 (29.1001, 4.0356) -> (29.2771, 4.0074)
  line L2452 (29.2771, 4.0074) -> (29.465, 3.9734)
  line L2453 (29.465, 3.9734) -> (29.6661, 3.9326)
  line L2454 (29.6661, 3.9326) -> (29.8774, 3.8852)
  line L2455 (29.8774, 3.8852) -> (30.0989, 3.8305)
  line L2456 (30.0989, 3.8305) -> (30.3325, 3.7677)
  line L2457 (30.3325, 3.7677) -> (30.5755, 3.6968)
  line L2458 (30.5755, 3.6968) -> (30.7866, 3.6308)
  arc A78 (30.8688, 2.8495) -> (30.7866, 3.6308) centre (0, 0) ccw
  line L2459 (30.8688, 2.8495) -> (30.676, 2.741)
  line L2460 (30.5004, -4.5761) -> (30.5788, -4.4112)
  line L2461 (30.5788, -4.4112) -> (30.6581, -4.2611)
  line L2462 (30.6581, -4.2611) -> (30.7375, -4.1249)
  line L2463 (30.7375, -4.1249) -> (30.8151, -4.0037)
  line L2464 (30.8151, -4.0037) -> (30.8928, -3.8929)
  line L2465 (30.8928, -3.8929) -> (30.9659, -3.7975)
  line L2466 (30.9659, -3.7975) -> (31.0351, -3.7146)
  line L2467 (31.0351, -3.7146) -> (31.0995, -3.6436)
  line L2468 (31.0995, -3.6436) -> (31.1577, -3.5847)
  line L2469 (31.1577, -3.5847) -> (31.2544, -3.498)
  line L2470 (31.2544, -3.498) -> (31.3364, -3.4375)
  line L2471 (31.3364, -3.4375) -> (31.3874, -3.4115)
  line L2472 (31.3874, -3.4115) -> (31.4881, -3.3539)
  line L2473 (31.4881, -3.3539) -> (31.5734, -3.2945)
  line L2474 (31.5734, -3.2945) -> (31.6432, -3.2343)
  line L2475 (31.6432, -3.2343) -> (31.6977, -3.1746)
  line L2476 (31.6977, -3.1746) -> (31.7371, -3.1165)
  line L2477 (31.7371, -3.1165) -> (31.7616, -3.0612)
  line L2478 (31.7616, -3.0612) -> (31.7684, -3.035)
  line L2479 (31.7684, -3.035) -> (31.7716, -3.0098)
  line L2480 (31.7716, -3.0098) -> (31.7712, -2.986)
  line L2481 (31.7712, -2.986) -> (31.7674, -2.9635)
  line L2482 (31.7674, -2.9635) -> (31.7578, -2.9376)
  line L2483 (31.7578, -2.9376) -> (31.6423, -2.7)
  line L2484 (31.6423, -2.7) -> (31.6076, -2.6235)
  line L2485 (31.6076, -2.6235) -> (31.5739, -2.5464)
  line L2486 (31.5739, -2.5464) -> (31.4746, -2.3016)
  line L2487 (31.4746, -2.3016) -> (31.4618, -2.2772)
  line L2488 (31.4618, -2.2772) -> (31.4477, -2.2593)
  line L2489 (31.4477, -2.2593) -> (31.4302, -2.2431)
  line L2490 (31.4302, -2.2431) -> (31.4094, -2.2286)
  line L2491 (31.4094, -2.2286) -> (31.3854, -2.2161)
  line L2492 (31.3854, -2.2161) -> (31.3279, -2.1973)
  line L2493 (31.3279, -2.1973) -> (31.2584, -2.1877)
  line L2494 (31.2584, -2.1877) -> (31.1775, -2.1883)
  line L2495 (31.1775, -2.1883) -> (31.0861, -2.1999)
  line L2496 (31.0861, -2.1999) -> (30.9848, -2.2234)
  line L2497 (30.9848, -2.2234) -> (30.8747, -2.2598)
  line L2498 (30.8747, -2.2598) -> (30.8212, -2.2803)
  line L2499 (30.8212, -2.2803) -> (30.7213, -2.3008)
  line L2500 (30.7213, -2.3008) -> (30.5923, -2.3146)
  line L2501 (30.5923, -2.3146) -> (30.5095, -2.3184)
  line L2502 (30.5095, -2.3184) -> (30.4137, -2.3188)
  line L2503 (30.4137, -2.3188) -> (30.3057, -2.3148)
  line L2504 (30.3057, -2.3148) -> (30.186, -2.3053)
  line L2505 (30.186, -2.3053) -> (30.0516, -2.2888)
  line L2506 (30.0516, -2.2888) -> (29.9096, -2.2654)
  line L2507 (29.9096, -2.2654) -> (29.7552, -2.2333)
  line L2508 (29.7552, -2.2333) -> (29.5907, -2.1918)
  line L2509 (29.5907, -2.1918) -> (29.4157, -2.1397)
  line L2510 (29.4157, -2.1397) -> (29.2602, -2.0868)
  arc A79 (29.1238, -1.4451) -> (29.2602, -2.0868) centre (37.5, 0) ccw
  line L2511 (29.1238, -1.4451) -> (29.2443, -1.3335)
  line L2512 (29.2443, -1.3335) -> (29.383, -1.2147)
  line L2513 (29.383, -1.2147) -> (29.5164, -1.1099)
  line L2514 (29.5164, -1.1099) -> (29.6444, -1.0178)
  line L2515 (29.6444, -1.0178) -> (29.7646, -0.9386)
  line L2516 (29.7646, -0.9386) -> (29.8807, -0.8689)
  line L2517 (29.8807, -0.8689) -> (29.9862, -0.8115)
  line L2518 (29.9862, -0.8115) -> (30.0832, -0.7639)
  line L2519 (30.0832, -0.7639) -> (30.1709, -0.7253)
  line L2520 (30.1709, -0.7253) -> (30.248, -0.6951)
  line L2521 (30.248, -0.6951) -> (30.3716, -0.6552)
  line L2522 (30.3716, -0.6552) -> (30.4711, -0.6334)
  line L2523 (30.4711, -0.6334) -> (30.5283, -0.6304)
  line L2524 (30.5283, -0.6304) -> (30.6437, -0.6187)
  line L2525 (30.6437, -0.6187) -> (30.7458, -0.5991)
  line L2526 (30.7458, -0.5991) -> (30.8341, -0.5725)
  line L2527 (30.8341, -0.5725) -> (30.9081, -0.5401)
  line L2528 (30.9081, -0.5401) -> (30.9677, -0.5031)
  line L2529 (30.9677, -0.5031) -> (31.0126, -0.4625)
  line L2530 (31.0126, -0.4625) -> (31.0295, -0.4413)
  line L2531 (31.0295, -0.4413) -> (31.0426, -0.4197)
  line L2532 (31.0426, -0.4197) -> (31.052, -0.3977)
  line L2533 (31.052, -0.3977) -> (31.0576, -0.3757)
  line L2534 (31.0576, -0.3757) -> (31.0594, -0.3481)
  line L2535 (31.0594, -0.3481) -> (31.0505, -0.0841)
  line L2536 (31.0505, -0.0841) -> (31.05, 0)
  line L2537 (31.05, 0) -> (31.0505, 0.0841)
  line L2538 (31.0505, 0.0841) -> (31.0594, 0.3481)
  line L2539 (31.0594, 0.3481) -> (31.0576, 0.3757)
  line L2540 (31.0576, 0.3757) -> (31.052, 0.3977)
  line L2541 (31.052, 0.3977) -> (31.0426, 0.4197)
  line L2542 (31.0426, 0.4197) -> (31.0295, 0.4413)
  line L2543 (31.0295, 0.4413) -> (31.0126, 0.4625)
  line L2544 (31.0126, 0.4625) -> (30.9677, 0.5031)
  line L2545 (30.9677, 0.5031) -> (30.9081, 0.5401)
  line L2546 (30.9081, 0.5401) -> (30.8341, 0.5725)
  line L2547 (30.8341, 0.5725) -> (30.7458, 0.5991)
  line L2548 (30.7458, 0.5991) -> (30.6437, 0.6187)
  line L2549 (30.6437, 0.6187) -> (30.5283, 0.6304)
  line L2550 (30.5283, 0.6304) -> (30.4711, 0.6334)
  line L2551 (30.4711, 0.6334) -> (30.3716, 0.6552)
  line L2552 (30.3716, 0.6552) -> (30.248, 0.6951)
  line L2553 (30.248, 0.6951) -> (30.1709, 0.7253)
  line L2554 (30.1709, 0.7253) -> (30.0832, 0.7639)
  line L2555 (30.0832, 0.7639) -> (29.9862, 0.8115)
  line L2556 (29.9862, 0.8115) -> (29.8807, 0.8689)
  line L2557 (29.8807, 0.8689) -> (29.7646, 0.9386)
  line L2558 (29.7646, 0.9386) -> (29.6444, 1.0178)
  line L2559 (29.6444, 1.0178) -> (29.5164, 1.1099)
  line L2560 (29.5164, 1.1099) -> (29.383, 1.2147)
  line L2561 (29.383, 1.2147) -> (29.2443, 1.3335)
  line L2562 (29.2443, 1.3335) -> (29.1238, 1.4451)
  arc A80 (29.2602, 2.0868) -> (29.1238, 1.4451) centre (37.5, 0) ccw
  line L2563 (29.2602, 2.0868) -> (29.4157, 2.1397)
  line L2564 (29.4157, 2.1397) -> (29.5907, 2.1918)
  line L2565 (29.5907, 2.1918) -> (29.7552, 2.2333)
  line L2566 (29.7552, 2.2333) -> (29.9096, 2.2654)
  line L2567 (29.9096, 2.2654) -> (30.0516, 2.2888)
  line L2568 (30.0516, 2.2888) -> (30.186, 2.3053)
  line L2569 (30.186, 2.3053) -> (30.3057, 2.3148)
  line L2570 (30.3057, 2.3148) -> (30.4137, 2.3188)
  line L2571 (30.4137, 2.3188) -> (30.5095, 2.3184)
  line L2572 (30.5095, 2.3184) -> (30.5923, 2.3146)
  line L2573 (30.5923, 2.3146) -> (30.7213, 2.3008)
  line L2574 (30.7213, 2.3008) -> (30.8212, 2.2803)
  line L2575 (30.8212, 2.2803) -> (30.8747, 2.2598)
  line L2576 (30.8747, 2.2598) -> (30.9848, 2.2234)
  line L2577 (30.9848, 2.2234) -> (31.0861, 2.1999)
  line L2578 (31.0861, 2.1999) -> (31.1775, 2.1883)
  line L2579 (31.1775, 2.1883) -> (31.2584, 2.1877)
  line L2580 (31.2584, 2.1877) -> (31.3279, 2.1973)
  line L2581 (31.3279, 2.1973) -> (31.3854, 2.2161)
  line L2582 (31.3854, 2.2161) -> (31.4094, 2.2286)
  line L2583 (31.4094, 2.2286) -> (31.4302, 2.2431)
  line L2584 (31.4302, 2.2431) -> (31.4477, 2.2593)
  line L2585 (31.4477, 2.2593) -> (31.4618, 2.2772)
  line L2586 (31.4618, 2.2772) -> (31.4746, 2.3016)
  line L2587 (31.4746, 2.3016) -> (31.5739, 2.5464)
  line L2588 (31.5739, 2.5464) -> (31.6076, 2.6235)
  line L2589 (31.6076, 2.6235) -> (31.6423, 2.7)
  line L2590 (31.6423, 2.7) -> (31.7578, 2.9376)
  line L2591 (31.7578, 2.9376) -> (31.7674, 2.9635)
  line L2592 (31.7674, 2.9635) -> (31.7712, 2.986)
  line L2593 (31.7712, 2.986) -> (31.7716, 3.0098)
  line L2594 (31.7716, 3.0098) -> (31.7684, 3.035)
  line L2595 (31.7684, 3.035) -> (31.7616, 3.0612)
  line L2596 (31.7616, 3.0612) -> (31.7371, 3.1165)
  line L2597 (31.7371, 3.1165) -> (31.6977, 3.1746)
  line L2598 (31.6977, 3.1746) -> (31.6432, 3.2343)
  line L2599 (31.6432, 3.2343) -> (31.5734, 3.2945)
  line L2600 (31.5734, 3.2945) -> (31.4881, 3.3539)
  line L2601 (31.4881, 3.3539) -> (31.3874, 3.4115)
  line L2602 (31.3874, 3.4115) -> (31.3364, 3.4375)
  line L2603 (31.3364, 3.4375) -> (31.2544, 3.498)
  line L2604 (31.2544, 3.498) -> (31.1577, 3.5847)
  line L2605 (31.1577, 3.5847) -> (31.0995, 3.6436)
  line L2606 (31.0995, 3.6436) -> (31.0351, 3.7146)
  line L2607 (31.0351, 3.7146) -> (30.9659, 3.7975)
  line L2608 (30.9659, 3.7975) -> (30.8928, 3.8929)
  line L2609 (30.8928, 3.8929) -> (30.8151, 4.0037)
  line L2610 (30.8151, 4.0037) -> (30.7375, 4.1249)
  line L2611 (30.7375, 4.1249) -> (30.6581, 4.2611)
  line L2612 (30.6581, 4.2611) -> (30.5788, 4.4112)
  line L2613 (30.5788, 4.4112) -> (30.5004, 4.5761)
  line L2614 (30.5004, 4.5761) -> (30.4357, 4.7271)
  arc A81 (30.8213, 5.2578) -> (30.4357, 4.7271) centre (37.5, 0) ccw
  line L2615 (30.8213, 5.2578) -> (30.9849, 5.243)
  line L2616 (30.9849, 5.243) -> (31.1659, 5.2193)
  line L2617 (31.1659, 5.2193) -> (31.3332, 5.1903)
  line L2618 (31.3332, 5.1903) -> (31.4872, 5.1568)
  line L2619 (31.4872, 5.1568) -> (31.6265, 5.1205)
  line L2620 (31.6265, 5.1205) -> (31.756, 5.0808)
  line L2621 (31.756, 5.0808) -> (31.8692, 5.0408)
  line L2622 (31.8692, 5.0408) -> (31.9695, 5.0006)
  line L2623 (31.9695, 5.0006) -> (32.0569, 4.9613)
  line L2624 (32.0569, 4.9613) -> (32.1309, 4.9241)
  line L2625 (32.1309, 4.9241) -> (32.2432, 4.859)
  line L2626 (32.2432, 4.859) -> (32.3261, 4.7997)
  line L2627 (32.3261, 4.7997) -> (32.3666, 4.7592)
  line L2628 (32.3666, 4.7592) -> (32.4524, 4.6812)
  line L2629 (32.4524, 4.6812) -> (32.5353, 4.6185)
  line L2630 (32.5353, 4.6185) -> (32.6142, 4.5707)
  line L2631 (32.6142, 4.5707) -> (32.6878, 4.5373)
  line L2632 (32.6878, 4.5373) -> (32.7552, 4.5178)
  line L2633 (32.7552, 4.5178) -> (32.8154, 4.5116)
  line L2634 (32.8154, 4.5116) -> (32.8424, 4.5132)
  line L2635 (32.8424, 4.5132) -> (32.8673, 4.518)
  line L2636 (32.8673, 4.518) -> (32.8899, 4.5257)
  line L2637 (32.8899, 4.5257) -> (32.9101, 4.5363)
  line L2638 (32.9101, 4.5363) -> (32.9317, 4.5534)
  line L2639 (32.9317, 4.5534) -> (33.122, 4.7366)
  line L2640 (33.122, 4.7366) -> (33.1841, 4.7933)
  line L2641 (33.1841, 4.7933) -> (33.2469, 4.8492)
  line L2642 (33.2469, 4.8492) -> (33.4491, 5.0192)
  line L2643 (33.4491, 5.0192) -> (33.4684, 5.039)
  line L2644 (33.4684, 5.039) -> (33.481, 5.0579)
  line L2645 (33.481, 5.0579) -> (33.491, 5.0796)
  line L2646 (33.491, 5.0796) -> (33.4983, 5.1038)
  line L2647 (33.4983, 5.1038) -> (33.5028, 5.1306)
  line L2648 (33.5028, 5.1306) -> (33.5029, 5.191)
  line L2649 (33.5029, 5.191) -> (33.4906, 5.2601)
  line L2650 (33.4906, 5.2601) -> (33.4651, 5.3368)
  line L2651 (33.4651, 5.3368) -> (33.4258, 5.4202)
  line L2652 (33.4258, 5.4202) -> (33.3721, 5.5092)
  line L2653 (33.3721, 5.5092) -> (33.3035, 5.6028)
  line L2654 (33.3035, 5.6028) -> (33.2674, 5.6473)
  line L2655 (33.2674, 5.6473) -> (33.2171, 5.7359)
  line L2656 (33.2171, 5.7359) -> (33.1641, 5.8544)
  line L2657 (33.1641, 5.8544) -> (33.1349, 5.9319)
  line L2658 (33.1349, 5.9319) -> (33.1049, 6.0229)
  line L2659 (33.1049, 6.0229) -> (33.0754, 6.1269)
  line L2660 (33.0754, 6.1269) -> (33.0474, 6.2437)
  line L2661 (33.0474, 6.2437) -> (33.0215, 6.3765)
  line L2662 (33.0215, 6.3765) -> (32.9999, 6.5189)
  line L2663 (32.9999, 6.5189) -> (32.9828, 6.6756)
  line L2664 (32.9828, 6.6756) -> (32.9714, 6.8449)
  line L2665 (32.9714, 6.8449) -> (32.9668, 7.0275)
  line L2666 (32.9668, 7.0275) -> (32.9691, 7.1917)
  arc A82 (33.5372, 7.5197) -> (32.9691, 7.1917) centre (37.5, 0) ccw
  line L2667 (33.5372, 7.5197) -> (33.6807, 7.4396)
  line L2668 (33.6807, 7.4396) -> (33.8364, 7.3444)
  line L2669 (33.8364, 7.3444) -> (33.9774, 7.2498)
  line L2670 (33.9774, 7.2498) -> (34.1045, 7.1566)
  line L2671 (34.1045, 7.1566) -> (34.217, 7.0668)
  line L2672 (34.217, 7.0668) -> (34.3191, 6.9779)
  line L2673 (34.3191, 6.9779) -> (34.4063, 6.8953)
  line L2674 (34.4063, 6.8953) -> (34.4815, 6.8178)
  line L2675 (34.4815, 6.8178) -> (34.5454, 6.7463)
  line L2676 (34.5454, 6.7463) -> (34.5979, 6.6822)
  line L2677 (34.5979, 6.6822) -> (34.674, 6.5771)
  line L2678 (34.674, 6.5771) -> (34.7256, 6.4892)
  line L2679 (34.7256, 6.4892) -> (34.7461, 6.4357)